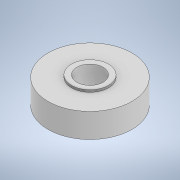
# Autodesk Inventor part: Load Cell
Saved by Autodesk Inventor 2021 (Build 250183000, 183)
## iProperties
Created: 2022-01-01
Part Number: Load Cell
Material: Generic
Document SubType Name: Modeling
Designer: Alex Clay
Density: 1 g/cm^3
Appearance: Default
Author: Alex Clay
Autodesk Inventor part; units mm, degrees
ref_plane "YZ Plane" through (0, 0, 0) normal (1, 0, 0) x (0, 1, 0)
ref_plane "XZ Plane" through (0, 0, 0) normal (0, 1, 0) x (-1, 0, 0)
ref_plane "XY Plane" through (0, 0, 0) normal (0, 0, 1) x (1, 0, 0)
sketch "Sketch1" plane through (0, 0, 0) normal (0, 0, 1) x (1, 0, 0)
  line L0 (7.9375, 16.002) -> (11.176, 16.002)
  line L1 (11.176, 16.002) -> (11.176, 14.732)
  line L2 (11.176, 14.732) -> (25.4, 14.732)
  line L3 (25.4, 14.732) -> (25.4, 0)
  line L4 (25.4, 0) -> (19.05, 0)
  line L5 (19.05, 0) -> (19.05, 1.27)
  line L6 (19.05, 1.27) -> (7.9375, 1.27)
  line L7 (7.9375, 1.27) -> (7.9375, 16.002)
  line L8 (0, -2.0008) -> (0, 23.5688) construction
  point P0 (0, 0)
  dimension "d0" = 25.4
  dimension "d1" = 19.05
  dimension "d2" = 7.9375
  dimension "d3" = 1.27
  dimension "d4" = 11.176
  dimension "d5" = 16.002
  dimension "d6" = 1.27
  constraints: 18 end point, 6 perpendicular, 2 point on line, 1 horizontal, 1 vertical
  measures "d0" distance from line of L8.start L3
  measures "d1" distance between parallel lines of L8 L5
  measures "d2" distance between parallel lines of L7 L8
  measures "d3" distance between parallel lines of L2 L0
  measures "d4" distance between parallel lines of L8 L1
  measures "d5" distance between parallel lines of L4 L0
  measures "d6" distance between parallel lines of L6 L4
revolve "Revolution1" add sketch "Sketch1" angle 360 about axis through (0, -2.0008, 0) along (0, 1, 0)
body "Solid1"
